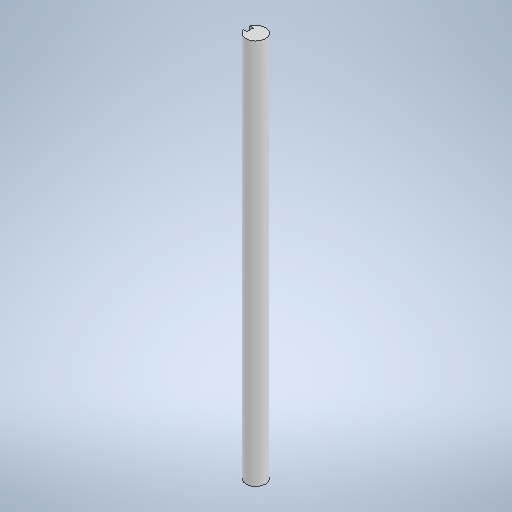
# Autodesk Inventor part: ShaftNut300mmV1
Saved by Autodesk Inventor 2025.1 (Build 291241000, 241)
## iProperties
Created: 2025-10-12
Part Number: ShaftNut300mmV1
Material: Generic
Document SubType Name: Modeling
Designer: jonas
Density: 1 g/cm^3
Appearance: Default
Author: jonas
Autodesk Inventor part; units mm, degrees
ref_plane "YZ Plane" through (0, 0, 0) normal (1, 0, 0) x (0, 1, 0)
ref_plane "XZ Plane" through (0, 0, 0) normal (0, 1, 0) x (-1, 0, 0)
ref_plane "XY Plane" through (0, 0, 0) normal (0, 0, 1) x (1, 0, 0)
sketch "Sketch1" plane through (0, 0, 0) normal (0, 1, 0) x (-1, 0, 0)
  line L0 (0, -8.4845) -> (0, 8.4845) construction
  line L1 (2.3645, 0) -> (-2.3645, 0) construction
  arc A0 (7.0711, 2.5) -> (7.0711, -2.5) centre (0, 0) ccw
  line L2 (7.0711, 2.5) -> (4.5, 2.5)
  line L3 (4.5, 2.5) -> (4.5, -2.5)
  line L4 (4.5, -2.5) -> (7.0711, -2.5)
  dimension "d0" = 15
  dimension "d1" = 4.5
  dimension "d3" = 5
  constraints: 10 end point, 2 coincident, 2 horizontal, 2 midpoint, 2 point on circle, 1 centre point, 1 parallel, 1 perpendicular, 1 vertical, 1 other
  measures "d0" diameter of A0
  measures "d1" distance between parallel lines of L0 L3
  measures "d3" distance of L2.end L3.end
extrude "Extrusion1" add sketch "Sketch1" along normal blind 300
body "Solid1"
